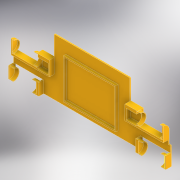
# Autodesk Inventor part: ChasisCircuiteria
Saved by Autodesk Inventor 2021 (Build 250183000, 183)
## iProperties
Created: 2024-02-22
Part Number: ChasisCircuiteria
Material: PLA
Document SubType Name: Modeling
Designer: Martin
Density: 1.27 g/cm^3
Appearance: PLA
Mass: 658.29 g
Surface Area: 2556.09 cm^2
Volume: 518.338 cm^3
Author: Martin
Autodesk Inventor part; units mm, degrees
ref_plane "YZ Plane" through (0, 0, 0) normal (1, 0, 0) x (0, 1, 0)
ref_plane "XZ Plane" through (0, 0, 0) normal (0, 1, 0) x (-1, 0, 0)
sketch "Sketch2" plane through (0, 0, 0) normal (1, 0, 0) x (0, 1, 0)
  arc A0 (-21.5, 0) -> (21.5, 0) centre (0, 0) ccw
  arc A1 (-23.5, 0) -> (23.5, 0) centre (0, 0) ccw
  line L0 (-23.5, 0) -> (23.5, 0)
  dimension "d0" = 43
  dimension "d1" = 47
  constraints: 4 point on circle, 2 centre point, 2 coincident, 2 end point, 2 point on line, 1 horizontal
  measures "d0" diameter of A0
  measures "d1" diameter of A1
extrude "SoporteCaderaAServo" add sketch "Sketch2" along normal blind 15 contours A0 L0 A1
sketch "Sketch3" plane through (15, 0, 0) normal (1, 0, 0) x (0, 0, -1)
  line L0 (8, 0) -> (8, 11.05)
  line L1 (8, 11.05) -> (18.5, 11.05)
  line L2 (18.5, 11.05) -> (18.5, -29.95)
  line L3 (18.5, -29.95) -> (8, -29.95)
  line L4 (8, -29.95) -> (8, 0)
  line L5 (8, 11.05) -> (0, 11.05)
  line L6 (0, 23.5) -> (0, 21.5) projected
  line L7 (0, 11.05) -> (0, 23.5)
  line L8 (0, 23.5) -> (18.5, 23.5)
  line L9 (18.5, 23.5) -> (23.5, 23.5)
  line L10 (23.5, 23.5) -> (23.5, -29.95)
  line L11 (23.5, -29.95) -> (23.5, -33.95)
  line L12 (23.5, -33.95) -> (0, -33.95)
  line L13 (0, -33.95) -> (0, -29.95)
  line L14 (0.7946, -29.95) -> (8, -29.95)
  line L15 (0.7946, -29.95) -> (0, -29.95)
  point P0 (0, 0)
  dimension "d4" = 11.05
  dimension "d5" = 10.5
  dimension "d6" = 41
  dimension "d7" = 8
  dimension "d9" = 4
  dimension "d31" = 5
  constraints: 30 end point, 8 perpendicular, 5 point on line, 2 horizontal, 1 collinear, 1 vertical
  measures "d4" distance of L0.start L0.end
  measures "d5" distance of L0.end L1.end
  measures "d6" distance of L1.end L2.end
  measures "d7" distance of point (0, 0) L0.start
  measures "d9" distance of L10.end L11.end
  measures "d31" distance between parallel lines of L10 L2
extrude "ProfundidadSErvo" add sketch "Sketch3" along normal blind 42 contours L5 L7 L6 L8 L9 L10 L11 L12 L13 L15 L14 L3 L2 L1
sketch "Sketch5" plane through (15, 0, 0) normal (-1, 0, 0) x (0, 0, 1)
  arc A0 (0, 23.5) -> (-23.5, 0) centre (0, 0) ccw projected
  line L0 (-18.5, 10.9545) -> (-18.5, -10.9545) projected
  line L1 (0, 11.05) -> (-18.4431, 11.05) projected
  arc A1 (-23.5, 0) -> (-18.5, -14.4914) centre (0, 0) ccw projected
  line L2 (-23.5, 23.5) -> (0, 23.5) projected
  line L3 (-23.5, -33.95) -> (-23.5, 0) projected
  line L4 (0, -33.95) -> (-23.5, -33.95) projected
  line L5 (0, -29.95) -> (0, -33.95) projected
  line L6 (-18.5, -29.95) -> (0, -29.95) projected
  line L7 (-18.5, -14.4914) -> (-18.5, -29.95) projected
  arc A2 (0, 23.5) -> (0, -23.5) centre (0, 0) ccw projected
  line L8 (0, -23.5) -> (0, -29.95)
  line L9 (-23.5, 0) -> (-23.5, 23.5) projected
  arc A3 (-18.5, 10.9545) -> (-18.5, -10.9545) centre (0, 0) ccw projected
  arc A4 (0, 21.5) -> (-18.4431, 11.05) centre (0, 0) ccw projected
  line L10 (0, 21.5) -> (0, 11.05) projected
  constraints: 2 end point, 1 vertical, 1 other
extrude "UnionCaderaServo" add sketch "Sketch5" along normal blind 4 contours A1 L7 L6 L5 L4 L3 | A0 L9 L2 | A2 L8 L6 L7
sketch "Sketch6" plane through (57, -33.95, -23.5) normal (0, -1, 0) x (1, 0, 0)
  line L0 (-46, 0) -> (0, 0) projected
  line L1 (0, 23.5) -> (0, 0) projected
  line L2 (-46, 23.5) -> (0, 23.5) projected
  line L3 (-46, 0) -> (-46, 23.5) projected
  point P0 (-57, 23.5)
extrude "AdicionParaRestringir" add sketch "Sketch6" along normal blind 15
sketch "Sketch7" plane through (11, 0, 0) normal (-1, 0, 0) x (0, 0, 1)
  line L0 (0, -23.5) -> (0, -48.95) projected
  line L1 (-23.5, 23.5) -> (-23.5, -48.95) projected
  line L2 (0, -26.4418) -> (-23.5, -26.4418)
  line L3 (-23.5, -26.4418) -> (-23.5, -48.95)
  line L4 (-23.5, -48.95) -> (0, -48.95)
  line L5 (0, -48.95) -> (0, -26.4418)
  point P0 (0, 0)
  point P1 (-23.5, -26.4418)
  constraints: 8 end point, 2 parallel, 1 horizontal, 1 perpendicular, 1 point on line
extrude "ExtrucionLongitudTubo" add sketch "Sketch7" along normal blind 98
sketch "Sketch8" plane through (-87, 0, 0) normal (-1, 0, 0) x (0, 0, 1)
  arc A0 (0, 23.5) -> (0, -23.5) centre (0, 0) ccw projected
  arc A1 (0, 21.5) -> (0, -21.5) centre (0, 0) ccw projected
  line L0 (0, 23.5) -> (0, 21.5) projected
  line L1 (0, -21.5) -> (0, -23.5) projected
extrude "SoporteTuboCadera" add sketch "Sketch8" against normal blind 8
sketch "Sketch9" plane through (-87, 0, 0) normal (-1, 0, 0) x (0, 0, 1)
  line L0 (-23.5, -26.4418) -> (0, -26.4418) projected
  line L1 (0, -23.5) -> (0, -26.4418) projected
  arc A0 (-23.5, 0) -> (0, -23.5) centre (0, 0) ccw projected
  arc A1 (0, 23.5) -> (-23.5, 0) centre (0, 0) ccw projected
  line L2 (0, 23.5) -> (-23.5, 23.5) projected
  line L3 (-23.5, 0) -> (-23.5, -26.4418) projected
  arc A2 (0, 21.5) -> (0, -21.5) centre (0, 0) ccw projected
  arc A3 (0, 23.5) -> (0, -23.5) centre (0, 0) ccw projected
  line L4 (0, -23.5) -> (0, -21.5) projected
  line L5 (0, 21.5) -> (0, 23.5) projected
  line L6 (0, -48.95) -> (0, -26.4418) projected
  line L7 (0, -26.4418) -> (-23.5, -26.4418) projected
  line L8 (-23.5, -26.4418) -> (-23.5, -48.95) projected
  line L9 (-23.5, -48.95) -> (0, -48.95) projected
  line L10 (0, -21.5) -> (0, 21.5)
  line L11 (-23.5, 23.5) -> (-23.5, 0) projected
  point P0 (-18.5, 10.9545)
  point P1 (-18.4431, 11.05)
  point P2 (-23.5, 0)
  point P3 (-22.5, 6.7823)
  point P4 (-23.5, 0)
  constraints: 2 end point, 1 vertical, 1 other
extrude "ParedTuboCadera" add sketch "Sketch9" along normal blind 4 contours L3 A0 L1 L0 | L0 L6 L9 L8 | A1 L5 A2 L4 A0 | A2 L10
sketch "Sketch10" plane through (57, 0, 0) normal (1, 0, 0) x (0, 0, -1)
  line L0 (0, -48.95) -> (0, 23.5) projected
  line L1 (0, -48.95) -> (19.5, -48.95)
  line L2 (19.5, -48.95) -> (19.5, -33.95)
  line L3 (19.5, -33.95) -> (0, -33.95)
  line L4 (0, -33.95) -> (0, -48.95)
  line L5 (23.5, 23.5) -> (23.5, -48.95) projected
  line L6 (18.5, -29.95) -> (0, -29.95) projected
  point P0 (0, 0)
  point P1 (0, -33.95)
  dimension "d24" = 4
  dimension "d25" = 4
  constraints: 8 end point, 2 parallel, 1 horizontal, 1 perpendicular
  measures "d24" distance between parallel lines of L2 L5
  measures "d25" distance between parallel lines of L6 L3
extrude "AhorrandoMaterial" cut sketch "Sketch10" against normal up to next
sketch "Sketch13" plane through (0, 0, 0) normal (1, 0, 0) x (0, 1, 0)
  arc A0 (-119.5, 0) -> (-76.5, 0) centre (-98, 0) ccw
  arc A1 (-121.5, 0) -> (-74.5, 0) centre (-98, 0) ccw
  line L0 (-119.5, 0) -> (-121.5, 0)
  line L1 (-76.5, 0) -> (-74.5, 0)
  point P0 (0, 0)
  dimension "d32" = 43
  dimension "d33" = 47
  constraints: 4 end point, 4 point on circle, 2 centre point, 2 coincident, 2 point on line, 1 horizontal
  measures "d32" diameter of A0
  measures "d33" diameter of A1
extrude "Soporte1Trasero" add sketch "Sketch13" along normal blind 15
sketch "Sketch14" plane through (15, 0, 0) normal (1, 0, 0) x (0, 0, -1)
  line L0 (0, -119.5) -> (0, -121.5) projected
  line L1 (0, -121.5) -> (23.5, -121.5)
  line L2 (23.5, -121.5) -> (23.5, -74.4078)
  line L3 (23.5, -74.4078) -> (0, -74.4078)
  line L4 (0, -74.4078) -> (0, -121.5)
  line L5 (23.5, 23.5) -> (23.5, -48.95) projected
  arc A0 (0, -121.5) -> (0, -74.5) centre (0, -98) ccw projected
  point P0 (0, 0)
  dimension "d41" = 0
  constraints: 8 end point, 2 parallel, 1 collinear, 1 horizontal, 1 perpendicular
  measures "d41" distance edge to line of A0 L2
extrude "Pared1SoporteTrasero" add sketch "Sketch14" along normal blind 4
sketch "Sketch15" plane through (15, -74.4078, 0) normal (0, 1, 0) x (1, 0, 0)
  line L0 (0, 23.5) -> (4, 23.5)
  line L1 (4, 23.5) -> (4, 19.5)
  line L2 (4, 19.5) -> (0, 19.5)
  line L3 (0, 19.5) -> (0, 23.5)
  point P0 (-15, 0)
  dimension "d38" = 4
  constraints: 8 end point, 2 parallel, 1 horizontal, 1 perpendicular
  measures "d38" distance of L0.end L1.end
extrude "UniendoTubos" add sketch "Sketch15" along normal up to surface (25.4578 mm away)
ref_plane "LongitudTrasero" through (-96.5, 0, 0) normal (-1, 0, 0) x (0, 0, 1)
sketch "Sketch17" plane through (-96.5, 0, 0) normal (-1, 0, 0) x (0, 0, 1)
  arc A0 (0, -76.5) -> (0, -119.5) centre (0, -98) ccw projected
  arc A1 (0, -74.5) -> (0, -121.5) centre (0, -98) ccw projected
  line L0 (0, -74.5) -> (0, -76.5) projected
  line L1 (0, -119.5) -> (0, -121.5) projected
  point P0 (0, 0)
extrude "Soporte2Trasero" add sketch "Sketch17" against normal blind 15
sketch "Sketch16" plane through (15, 0, 0) normal (-1, 0, 0) x (0, 0, 1)
  line L0 (-19.5, -74.4078) -> (0, -74.4078) projected
  line L1 (-23.5, -121.5) -> (-23.5, -48.95) projected
  line L2 (-19.5, -48.95) -> (-23.5, -48.95)
  line L3 (-23.5, -48.95) -> (-23.5, -74.4078)
  line L4 (-23.5, -74.4078) -> (-19.5, -74.4078)
  line L5 (-19.5, -74.4078) -> (-19.5, -48.95)
  point P0 (0, 0)
  constraints: 8 end point, 2 parallel, 1 horizontal, 1 perpendicular, 1 point on line
extrude "ExpandiendoUnion" add sketch "Sketch16" along normal up to surface (111.5 mm away)
sketch "Sketch18" plane through (-96.5, 0, 0) normal (-1, 0, 0) x (0, 0, 1)
  line L0 (0, -74.5) -> (0, -76.5) projected
  line L1 (0, -121.5) -> (-23.5, -121.5) projected
  line L2 (0, -74.5) -> (-23.5, -74.5)
  line L3 (-23.5, -74.5) -> (-23.5, -121.5)
  line L4 (-23.5, -121.5) -> (0, -121.5)
  line L5 (0, -121.5) -> (0, -74.5)
  line L6 (-19.5, -74.4078) -> (-19.5, -48.95) projected
  line L7 (-19.5, -48.95) -> (-23.5, -48.95)
  line L8 (-23.5, -48.95) -> (-23.5, -74.5)
  line L9 (-23.5, -74.5) -> (-19.5, -74.5)
  line L10 (-19.5, -74.5) -> (-19.5, -48.95)
  point P0 (0, 0)
  constraints: 16 end point, 4 parallel, 2 horizontal, 2 perpendicular
extrude "Pared2SoporteTrasero" add sketch "Sketch18" along normal blind 4
sketch "Sketch21" plane through (19, 0, 0) normal (1, 0, 0) x (0, 0, -1)
  line L0 (0, -74.4078) -> (0, -121.5) projected
  line L1 (0, -121.5) -> (23.5, -121.5) projected
  line L2 (23.5, -121.5) -> (23.5, -48.95) projected
  line L3 (19.5, -48.95) -> (23.5, -48.95) projected
  line L4 (19.5, -74.4078) -> (19.5, -48.95) projected
  line L5 (19.5, -74.4078) -> (0, -74.4078) projected
  line L6 (19.5, -48.95) -> (23.5, -48.95)
  line L7 (23.5, -48.95) -> (23.5, -121.5)
  line L8 (23.5, -121.5) -> (19.5, -121.5)
  line L9 (19.5, -121.5) -> (19.5, -48.95)
  point P0 (0, 0)
  constraints: 8 end point, 2 parallel, 1 horizontal, 1 perpendicular
sketch "Sketch22" plane through (57, 0, 0) normal (1, 0, 0) x (0, 0, -1)
  line L0 (19.5, -33.95) -> (19.5, -48.95) projected
  line L1 (23.5, -48.95) -> (19.5, -48.95) projected
  line L2 (23.5, 23.5) -> (23.5, -48.95) projected
  line L3 (23.5, 23.5) -> (0, 23.5) projected
  line L4 (0, 23.5) -> (0, 11.05) projected
  line L5 (0, 11.05) -> (18.5, 11.05) projected
  line L6 (18.5, 11.05) -> (18.5, -29.95) projected
  line L7 (18.5, -29.95) -> (0, -29.95) projected
  line L8 (0, -29.95) -> (0, -33.95) projected
  line L9 (0, -33.95) -> (19.5, -33.95) projected
  line L10 (0, -33.95) -> (23.5, -33.95)
  line L11 (23.5, -33.95) -> (23.5, 23.5)
  line L12 (23.5, 23.5) -> (0, 23.5)
  line L13 (0, 23.5) -> (0, -33.95)
  point P0 (0, 0)
  constraints: 8 end point, 2 parallel, 1 horizontal, 1 perpendicular
extrude "Extrusion17" add sketch "Sketch22" along normal blind 4 contours L9 L8 L7 L6 L5 L4 L3 L2 L10 | L13 L5 L6 L7
extrude "Extrusion18" add sketch "Sketch21" along normal up to surface (42 mm away) contours L4 L3 L2 L1 L9
sketch "Sketch23" plane through (57, 0, 0) normal (1, 0, 0) x (0, 0, -1)
  line L0 (23.5, -33.95) -> (19.5, -33.95) projected
  line L1 (19.5, -33.95) -> (19.5, -48.95) projected
  line L2 (23.5, -48.95) -> (19.5, -48.95) projected
  line L3 (23.5, -33.95) -> (23.5, -48.95) projected
  point P0 (0, 0)
extrude "Extrusion19" add sketch "Sketch23" along normal up to surface (4 mm away)
sketch "Sketch24" plane through (61, 0, 0) normal (1, 0, 0) x (0, 0, -1)
  line L0 (0, -33.95) -> (19.5, -33.95) projected
  line L1 (19.5, -121.5) -> (19.5, -33.95) projected
  line L2 (23.5, -121.5) -> (19.5, -121.5) projected
  line L3 (23.5, 23.5) -> (23.5, -121.5) projected
  line L4 (23.5, 23.5) -> (0, 23.5) projected
  line L5 (0, 23.5) -> (0, -33.95) projected
  line L6 (23.5, -121.5) -> (19.5, -121.5)
  line L7 (19.5, -121.5) -> (19.5, 23.5)
  line L8 (19.5, 23.5) -> (23.5, 23.5)
  line L9 (23.5, 23.5) -> (23.5, -121.5)
  point P0 (0, 0)
  constraints: 8 end point, 2 parallel, 1 horizontal, 1 perpendicular, 1 point on line
extrude "Extrusion20" add sketch "Sketch24" along normal blind 50 contours L7 L4 L3 L2 L1
sketch "Sketch26" plane through (11, 23.5, 0) normal (0, 1, 0) x (1, 0, 0)
  line L0 (0, 0) -> (50, 0) projected
  line L1 (50, 19.5) -> (50, 0) projected
  line L2 (50, 19.5) -> (100, 19.5) projected
  line L3 (100, 23.5) -> (100, 19.5) projected
  line L4 (0, 23.5) -> (100, 23.5) projected
  line L5 (0, 0) -> (0, 23.5) projected
  line L6 (100, 23.5) -> (50, 23.5)
  line L7 (50, 23.5) -> (50, 19.5)
  line L8 (50, 19.5) -> (100, 19.5)
  line L9 (100, 19.5) -> (100, 23.5)
  point P0 (-11, 0)
  constraints: 8 end point, 2 parallel, 1 horizontal, 1 perpendicular
extrude "Extrusion21" add sketch "Sketch26" along normal blind 80 contours L7 L4 L3 L2
sketch "Sketch28" plane through (19, -121.5, -19.5) normal (0, 0, 1) x (1, 0, 0)
  line L0 (-110, 72.55) -> (-110, 87.55) projected
  line L1 (-115.5, 47) -> (-119.5, 47) projected
  line L2 (-115.5, 47) -> (-115.5, 47.0922) projected
  line L3 (-4, 47.0922) -> (-115.5, 47.0922) projected
  line L4 (0, 47.0922) -> (-4, 47.0922) projected
  line L5 (0, 0) -> (0, 47.0922) projected
  line L6 (0, 0) -> (92, 0) projected
  line L7 (92, 0) -> (92, 225) projected
  line L8 (42, 225) -> (92, 225) projected
  line L9 (42, 145) -> (42, 225) projected
  line L10 (42, 87.55) -> (42, 145) projected
  line L11 (42, 87.55) -> (-110, 87.55) projected
  line L12 (92, 0) -> (92, 225) projected
  line L13 (92, 175) -> (88, 175)
  line L14 (88, 175) -> (88, 25)
  line L15 (88, 25) -> (92, 25)
  line L16 (92, 25) -> (92, 175)
  line L17 (-110, 72.55) -> (-119.5, 72.55) projected
  line L18 (-119.5, 47) -> (-119.5, 72.55) projected
  point P0 (-19, 121.5)
  point P1 (92, 25)
  dimension "d59" = 4
  dimension "d60" = 150
  dimension "d73" = 25
  constraints: 8 end point, 2 parallel, 1 horizontal, 1 perpendicular, 1 point on line
  measures "d59" distance of L15.end L14.end
  measures "d60" distance of L14.end L13.end
  measures "d73" distance between parallel lines of L6 L15
sketch "Sketch29" plane through (111, 0, 0) normal (1, 0, 0) x (0, 0, -1)
  line L0 (19.5, -121.5) -> (19.5, 103.5) projected
  line L1 (19.5, -121.5) -> (23.5, -121.5) projected
  line L2 (23.5, -121.5) -> (23.5, 103.5) projected
  line L3 (19.5, 103.5) -> (23.5, 103.5) projected
  point P0 (0, 0)
extrude "Extrusion22" add sketch "Sketch28" along normal blind 10 contours L7 L15 L14 L13
extrude "Extrusion23" add sketch "Sketch29" along normal blind 100
sketch "Sketch30" plane through (19, -121.5, -19.5) normal (0, 0, 1) x (1, 0, 0)
  line L0 (88, 25) -> (92, 25) projected
  line L1 (92, 25) -> (92, 175) projected
  line L2 (92, 175) -> (88, 175) projected
  line L3 (88, 175) -> (88, 25) projected
  line L4 (92, 25) -> (88, 25) projected
  line L5 (88, 25) -> (88, 175) projected
  line L6 (88, 175) -> (92, 175) projected
  line L7 (92, 25) -> (92, 175) projected
  line L8 (0, 0) -> (192, 0) projected
  line L9 (192, 225) -> (192, 0) projected
  line L10 (42, 225) -> (192, 225) projected
  line L11 (42, 145) -> (42, 225) projected
  line L12 (42, 87.55) -> (42, 145) projected
  line L13 (42, 87.55) -> (-110, 87.55) projected
  line L14 (-110, 72.55) -> (-110, 87.55) projected
  line L15 (-115.5, 47) -> (-119.5, 47) projected
  line L16 (-115.5, 47) -> (-115.5, 47.0922) projected
  line L17 (-4, 47.0922) -> (-115.5, 47.0922) projected
  line L18 (0, 47.0922) -> (-4, 47.0922) projected
  line L19 (0, 0) -> (0, 47.0922) projected
  line L20 (192, 0) -> (192, 225) projected
  line L21 (88, 175) -> (192, 175)
  line L22 (192, 175) -> (192, 179)
  line L23 (192, 179) -> (88, 179)
  line L24 (88, 179) -> (88, 175)
  line L25 (88, 25) -> (192, 25)
  line L26 (192, 25) -> (192, 21)
  line L27 (192, 21) -> (88, 21)
  line L28 (88, 21) -> (88, 25)
  line L29 (-110, 72.55) -> (-119.5, 72.55) projected
  line L30 (-119.5, 47) -> (-119.5, 72.55) projected
  point P0 (-19, 121.5)
  point P1 (192, 179)
  dimension "d65" = 4
  dimension "d66" = 4
  constraints: 16 end point, 4 parallel, 2 horizontal, 2 perpendicular, 2 point on line
  measures "d65" distance of L22.end L21.end
  measures "d66" distance of L25.end L26.end
extrude "Extrusion24" add sketch "Sketch30" along normal up to surface (10 mm away) contours L0 L25 L9 L27 L28 | L24 L23 L9 L21 L2
sketch "Sketch31" plane through (15, 0, 0) normal (-1, 0, 0) x (0, 0, 1)
  arc A0 (0, -76.5) -> (0, -119.5) centre (0, -98) ccw projected
  line L0 (0, -121.5) -> (0, -74.5) projected
  point P0 (0, 0)
extrude "Extrusion25" add sketch "Sketch31" along normal blind 6.5
sketch "Sketch32" plane through (0, 0, 0) normal (-1, 0, 0) x (0, 0, 1)
  arc A0 (0, -76.5) -> (0, -119.5) centre (0, -98) ccw projected
  arc A1 (0, -74.5) -> (-23.5, -98) centre (0, -98) ccw projected
  arc A2 (-23.5, -98) -> (0, -121.5) centre (0, -98) ccw projected
  line L0 (0, -121.5) -> (0, -74.5) projected
  point P0 (0, 0)
extrude "Extrusion26" add sketch "Sketch32" along normal blind 6.5 contours A0 L0 A2 A1
mirror "Mirror1" about plane through (211, -9, -21.5) normal (1, 0, 0) of "Extrusion19", "Extrusion20", "Extrusion26", "Extrusion22", "Extrusion23", "Extrusion24", "Extrusion25", "Extrusion21", "Extrusion18", "Pared2SoporteTrasero", "ExpandiendoUnion", "Soporte2Trasero", "Pared1SoporteTrasero", "Soporte1Trasero", "AhorrandoMaterial", "ParedTuboCadera", "ExtrucionLongitudTubo", "SoporteTuboCadera", "AdicionParaRestringir", "UnionCaderaServo", "ProfundidadSErvo", "SoporteCaderaAServo", "UniendoTubos", "Extrusion17"
ref_plane "Work Plane2" through (518.5, 0, 0) normal (-1, 0, 0) x (0, 0, 1)
body "Solid1"
